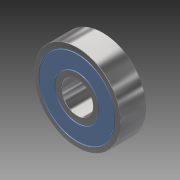
# Autodesk Inventor part: fc16-062
Saved by Autodesk Inventor 2016 SP1 (Build 200210100, 210)
## iProperties
Category: Bearing
Company: Autodesk Inc.
Created: 2015-12-03
Part Number: fc16-062
Material: Stainless Steel, 440C
Document SubType Name: Modeling
Designer: Autodesk Inc.
Density: 7.75 g/cm^3
Appearance: Steel - Polished
Catalog Web Link: http://www.shusterbearings.com/shopexd.asp?id=98
Vendor: Shuster
Author: Autodesk Inc.
Keywords: FIRSTChoice
Autodesk Inventor part; units mm, degrees
ref_plane "YZ Plane" through (0, 0, 0) normal (1, 0, 0) x (0, 1, 0)
ref_plane "XZ Plane" through (0, 0, 0) normal (0, 1, 0) x (-1, 0, 0)
sketch "Sketch1" plane through (0, 0, 0) normal (0, 1, 0) x (-1, 0, 0)
  circle A0 centre (0, 0) radius 8.5
  circle A1 centre (0, 0) radius 23.5
  dimension "d0" = 17
  dimension "d1" = 47
  constraints: 2 centre point, 2 coincident
  measures "d0" diameter of A0
  measures "d1" diameter of A1
extrude "Extrusion1" add sketch "Sketch1" against normal blind 14
fillet "Fillet1" radius 0.3 4 edges at (23.5, 0, 0) (23.5, -14, 0) (8.5, 0, 0) (8.5, -14, 0)
sketch "Sketch2" plane through (0, 0, 0) normal (1, 0, 0) x (0, 1, 0)
  line L0 (-14, -23.2) -> (-14, 23.2) projected
  line L1 (-0.3, 23.5) -> (-13.7, 23.5) projected
  circle A0 centre (-14, 20.4966) radius 0.3168
  circle A1 centre (-14, 11.8967) radius 0.3168
  line L2 (-19.5802, 0) -> (3.2634, 0) projected
  point P0 (0, 0)
  constraints: 2 centre point, 2 point on line, 1 equal radius
revolve "Revolution1" cut sketch "Sketch2" angle 360 about axis through (0, -10, 0) along (0, 1, 0)
ref_plane "Work Plane1" through (0, -7, 0) normal (0, 1, 0) x (1, 0, 0)
mirror "Mirror1" about plane through (0, -7, 0) normal (0, 1, 0) of "Revolution1"
body "Solid1"
